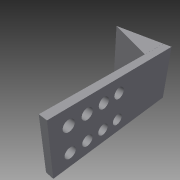
# Autodesk Inventor part: Mount for camera
Saved by Autodesk Inventor 2015 (Build 190159000, 159)
## iProperties
Created: 2018-11-12
Part Number: Mount for camera
Material: Типовые
Document SubType Name: Modeling
Designer: kostya
Density: 1 g/cm^3
Appearance: По умолчанию
Author: kostya
Autodesk Inventor part; units mm, degrees
ref_plane "YZ Plane" through (0, 0, 0) normal (1, 0, 0) x (0, 1, 0)
ref_plane "XZ Plane" through (0, 0, 0) normal (0, 1, 0) x (-1, 0, 0)
ref_plane "XY Plane" through (0, 0, 0) normal (0, 0, 1) x (1, 0, 0)
sketch "Эскиз5" plane through (0, 0, 0) normal (0, 0, 1) x (1, 0, 0)
  line L0 (0, 0) -> (20, 0)
  line L1 (20, 0) -> (20, -10)
  line L2 (20, -10) -> (0, 0)
  dimension "d14" = 20
  dimension "d15" = 10
  constraints: 6 end point, 1 horizontal, 1 perpendicular
  measures "d14" distance of L0.start L0.end
  measures "d15" distance of L0.end L1.end
extrude "Выдавливание5" add sketch "Эскиз5" against normal blind 20
sketch "Эскиз6" plane through (0, 0, 0) normal (0, 0, 1) x (1, 0, 0)
  line L0 (20.0268, 0) -> (23.0268, 0)
  line L1 (23.0268, 0) -> (23.0268, -50)
  line L2 (23.0268, -50) -> (20.0268, -50)
  line L3 (20.0268, -50) -> (20.0268, 0)
  point P0 (0, 0)
  dimension "d18" = 3
  dimension "d19" = 50
  constraints: 8 end point, 2 parallel, 1 horizontal, 1 perpendicular
  measures "d18" distance of L1.end L2.end
  measures "d19" distance of L0.end L1.end
extrude "Выдавливание6" add sketch "Эскиз6" against normal blind 20
sketch "Эскиз7" plane through (23.0268, -50, 0) normal (1, 0, 0) x (0, 0, -1)
  line L0 (0, 50) -> (0, 0) projected
  line L1 (0, 0) -> (20, 0) projected
  line L2 (20, 50) -> (20, 0) projected
  line L3 (0, 50) -> (20, 50) projected
  line L4 (10, 50) -> (10.622, 0) construction
  line L5 (20, 50) -> (20, 0) construction
  line L6 (20, 25) -> (0, 25) construction
  line L7 (20, 25) -> (20, 0) construction
  line L8 (20, 12.5) -> (0, 12.5) construction
  line L9 (0, -0.1321) -> (0, 25) construction
  line L10 (0, 50) -> (0, 25) construction
  line L11 (0, 25) -> (0, 50) construction
  line L12 (0, 50) -> (0, 25) construction
  line L13 (0, 37.5) -> (20, 37.5) construction
  line L14 (0, 50) -> (10, 50) construction
  line L15 (20, 50) -> (10, 50) construction
  line L16 (0, 50) -> (10, 50) construction
  line L17 (5, 50) -> (5.6228, 0) construction
  line L18 (20, 50) -> (10, 50) construction
  line L19 (15, 50) -> (15, 0) construction
  circle A0 centre (5.4671, 12.5) radius 2
  circle A1 centre (15, 12.5) radius 2
  circle A2 centre (15, 25) radius 2
  circle A3 centre (5.3114, 25) radius 2.0002
  line L20 (0, 12.5) -> (0, 0) construction
  line L21 (0, 50) -> (0, 0) construction
  line L22 (0, -0.1321) -> (0, 12.5) construction
  line L23 (0, 6.1839) -> (20, 6.1839) construction
  circle A4 centre (5.5458, 6.1839) radius 2
  circle A5 centre (15, 6.1839) radius 2
  line L24 (0, 25) -> (0, 12.5)
  line L25 (0, 18.75) -> (20, 18.75) construction
  circle A6 centre (5.3892, 18.75) radius 2
  circle A7 centre (15, 18.75) radius 2
  line L26 (0, 37.5) -> (0, 25)
  line L27 (0, 31.25) -> (20, 31.25) construction
  dimension "d22" = 4
  dimension "d23" = 4
  dimension "d27" = 4
  dimension "d28" = 4
  dimension "d29" = 4
  constraints: 44 end point, 22 point on line, 12 midpoint, 11 collinear, 8 centre point, 6 perpendicular, 1 parallel, 1 vertical
  measures "d22" diameter of A0
  measures "d23" diameter of A2
  measures "d27" diameter of A4
  measures "d28" diameter of A5
  measures "d29" diameter of A6
extrude "Выдавливание7" cut sketch "Эскиз7" against normal blind 20 contours A0 | A1 | A2 | A3 | A4 | A5 | A6 | A7
